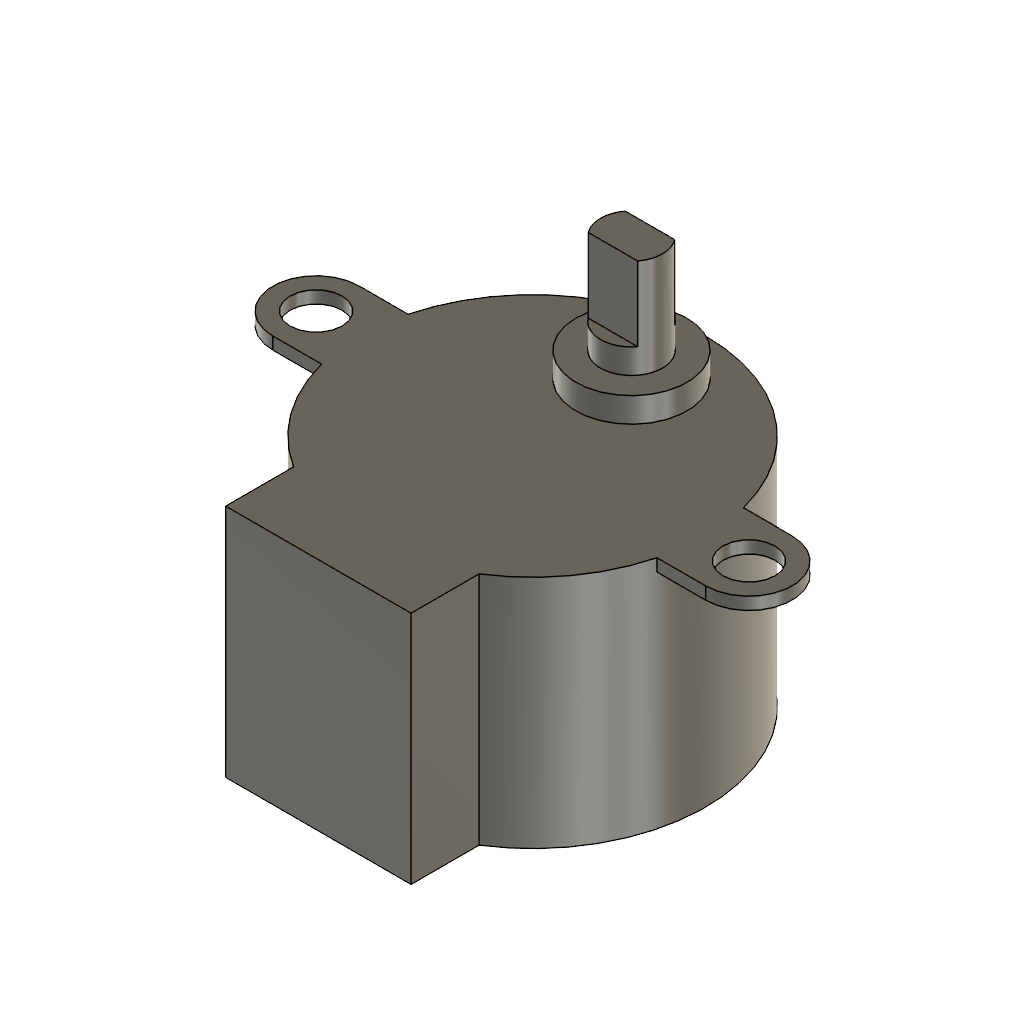
03 - 28BYJ-48 STEPPER MOTOR (Autodesk Fusion 360 design; units mm, degrees)
Autodesk Fusion 360 part; units mm, degrees
note: some values were not read from the file. Set by a fixed rule: which sketch regions a step uses.
sketch "01 - 28BYJ-48 STEPPER MOTOR BASE SKETCH" plane through (0, 0, 0) normal (0, 0, 1) x (1, 0, 0) in component "01 - 28BYJ-48 STEPPER MOTOR BASE"
  line L0 (-17.5, 0) -> (17.5, 0) construction
  circle A0 centre (-17.5, 0) radius 2.1
  circle A1 centre (17.5, 0) radius 2.1
  arc A2 (-17.5, 3.5) -> (-17.5, -3.5) centre (-17.5, 0) ccw
  arc A3 (17.5, -3.5) -> (17.5, 3.5) centre (17.5, 0) ccw
  line L1 (-17.5, 3.5) -> (-13.5554, 3.5)
  line L2 (13.5554, 3.5) -> (17.5, 3.5)
  line L3 (-17.5, -3.5) -> (-13.5554, -3.5)
  line L4 (13.5554, -3.5) -> (17.5, -3.5)
  line L5 (-7.5, -17.3216) -> (7.5, -17.3216)
  line L6 (7.5, -17.3216) -> (7.5, -11.8216)
  line L7 (-7.5, -17.3216) -> (-7.5, -11.8216)
  line L8 (0, 0) -> (0, 8)
  circle A4 centre (0, 8) radius 4.5
  line L9 (-7.5, -11.8216) -> (-7.5, 0) construction
  line L10 (7.5, -11.8216) -> (7.5, 0) construction
  line L11 (0, -17.3216) -> (0, 0) construction
  line L12 (0, 8) -> (0, 14) construction
  arc A5 (7.5, -11.8216) -> (-7.5, -11.8216) centre (0, 0) ccw
  dimension "d1" = 28
  dimension "d2" = 35
  dimension "d3" = 4.2
  dimension "d4" = 7
  dimension "d5" = 4.2
  dimension "d6" = 7
  dimension "d8" = 15
  dimension "d9" = 8
  dimension "d10" = 9
  dimension "d21" = 5.5
  dimension "d23" = 5.5
  dimension "d36" = 6
  dimension "d37" = 25.3216
  constraint coincident L8.start L11.end
  constraint horizontal L0
  constraint midpoint L8.start L0
  constraint coincident L0.start A0.centre
  constraint concentric A0 A2
  constraint coincident L0.end A1.centre
  constraint concentric A1 A3
  constraint tangent A3 L2
  constraint tangent A2 L1
  constraint tangent A3 L4
  constraint tangent A2 L3
  constraint coincident L1.end A5
  constraint coincident L2.start A5
  constraint collinear L1 L2
  constraint coincident L3.end A5
  constraint coincident L4.start A5
  constraint collinear L3 L4
  constraint perpendicular L5 L6
  constraint perpendicular L5 L7
  constraint perpendicular L0 L8
  constraint coincident L8.end A4.centre
  constraint coincident L0 L9.end
  constraint perpendicular L0 L9
  constraint coincident L0 L10.end
  constraint perpendicular L0 L10
  constraint midpoint L5 L11.start
  constraint perpendicular L0 L11
  constraint coincident L12.end A5
  constraint perpendicular L12 A5
  measures "d1" diameter of A5
  measures "d2" distance of L0.start L0.end
  measures "d3" diameter of A0
  measures "d4" diameter of A2
  measures "d5" diameter of A1
  measures "d6" diameter of A3
  measures "d8" distance of L5.start L5.end
  measures "d9" distance of L8.start L8.end
  measures "d10" diameter of A4
  measures "d21" distance of L5.end L6.end
  measures "d23" distance of L5.start L7.end
  measures "d36" distance of L8.end L12.end
  measures "d37" distance of L5 L8.end
extrude "Extrude1" add sketch "01 - 28BYJ-48 STEPPER MOTOR BASE SKETCH" against normal blind 19 contours L5 L6 L7 A5 | A4 makes body 1 in component "01 - 28BYJ-48 STEPPER MOTOR BASE"
extrude "Extrude2" add sketch "01 - 28BYJ-48 STEPPER MOTOR BASE SKETCH" along normal blind 2 contours A4 bodies 1 in component "01 - 28BYJ-48 STEPPER MOTOR BASE"
extrude "Extrude3" add sketch "01 - 28BYJ-48 STEPPER MOTOR BASE SKETCH" against normal blind 1 contours A2 L1 L3 A5 | A3 L2 L4 A5 bodies 1 in component "01 - 28BYJ-48 STEPPER MOTOR BASE"
extrude "Extrude4" add sketch "01 - 28BYJ-48 STEPPER MOTOR BASE SKETCH" against normal blind 16 contours L5 L6 L7 A5 | A4 bodies 1 in component "01 - 28BYJ-48 STEPPER MOTOR BASE"
sketch "02 - 28BYJ-48 STEPPER MOTOR SHAFT SKETCH" plane through (0, 0, 2) normal (0, 0, 1) x (-1, 0, 0) in component "02 - 28BYJ-48 STEPPER MOTOR SHAFT"
  circle A0 centre (0, -8) radius 4.5
  circle A1 centre (0, -8) radius 2.5
  line L0 (2, -9.5) -> (-2, -9.5)
  line L1 (2, -6.5) -> (-2, -6.5)
  dimension "d24" = 5
  dimension "d25" = 3
  constraint concentric A0 A1
  constraint coincident A1 L0.start
  constraint coincident A1 L0.end
  constraint horizontal L0
  constraint coincident A1 L1.start
  constraint coincident A1 L1.end
  constraint horizontal L1
  constraint equal L0 L1
  measures "d24" diameter of A1
  measures "d25" distance of L0 L1
extrude "Extrude1'" add sketch "02 - 28BYJ-48 STEPPER MOTOR SHAFT SKETCH" along normal blind 2 separate body contours A1 L1 | A1 L0 makes body 2 at (-1.9264, 6.4066, 2.6667) makes body 3 at (0.9832, 10.2985, 3.3333) in component "02 - 28BYJ-48 STEPPER MOTOR SHAFT"
extrude "Extrude2'" add sketch "02 - 28BYJ-48 STEPPER MOTOR SHAFT SKETCH" along normal blind 8 contours A1 L0 L1 bodies 2 3 in component "02 - 28BYJ-48 STEPPER MOTOR SHAFT"
component "01 - 28BYJ-48 STEPPER MOTOR BASE" placed x (1, 0, 0) y (0, 1, 0) z (0, 0, 1) at (0, 0, 0)
component "02 - 28BYJ-48 STEPPER MOTOR SHAFT" placed x (1, 0, 0) y (0, 1, 0) z (0, 0, 1) at (0, 0, 0)
named bodies: "01 - 28BYJ-48 STEPPER MOTOR BASE", "02 - 28BYJ-48 STEPPER MOTOR SHAFT"
